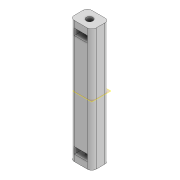
# Autodesk Inventor part: TopBottomConnector
Saved by Autodesk Inventor 2022 (Build 260153000, 153)
## iProperties
Created: 2022-10-26
Part Number: TopBottomConnector
Material: Generic
Document SubType Name: Modeling
Designer: MVeszpremi
Density: 1 g/cm^3
Appearance: Default
Author: MVeszpremi
Autodesk Inventor part; units mm, degrees
ref_plane "YZ Plane" through (0, 0, 0) normal (1, 0, 0) x (0, 1, 0)
ref_plane "XZ Plane" through (0, 0, 0) normal (0, 1, 0) x (-1, 0, 0)
ref_plane "XY Plane" through (0, 0, 0) normal (0, 0, 1) x (1, 0, 0)
sketch "Sketch1" plane through (0, 0, 0) normal (0, 1, 0) x (-1, 0, 0)
  line L0 (0, 0) -> (10, 0)
  line L1 (10, 0) -> (10, -8)
  line L2 (10, -8) -> (0, -8)
  line L3 (0, -8) -> (0, 0)
  circle A0 centre (5, -4) radius 1.5
  dimension "d0" = 10
  dimension "d1" = 8
  dimension "d2" = 3
  dimension "d11" = 5
  dimension "d12" = 4
  constraints: 8 end point, 2 parallel, 1 centre point, 1 horizontal, 1 perpendicular
  measures "d0" distance of L1.end L2.end
  measures "d1" distance of L0.end L1.end
  measures "d2" diameter of A0
  measures "d11" distance from line of A0.centre L1
  measures "d12" distance from line of L2 A0.centre
extrude "Extrusion1" add sketch "Sketch1" along normal blind 56
sketch "Sketch2" plane through (-10, 0, 0) normal (0, 0, 1) x (1, 0, 0)
  line L0 (2, 6) -> (8, 6)
  line L1 (8, 6) -> (8, 3)
  line L2 (8, 3) -> (2, 3)
  line L3 (2, 3) -> (2, 6)
  line L4 (0, 0) -> (0, 56) projected
  line L5 (0, 0) -> (10, 0) projected
  dimension "d5" = 6
  dimension "d6" = 2
  dimension "d7" = 3
  dimension "d8" = 3
  constraints: 8 end point, 2 parallel, 1 horizontal, 1 perpendicular
  measures "d5" distance of L0.start L0.end
  measures "d6" distance between parallel lines of L4 L3
  measures "d7" distance between parallel lines of L5 L2
  measures "d8" distance of L0.end L1.end
extrude "Extrusion2" cut sketch "Sketch2" against normal blind 61
ref_plane "Work Plane1" through (0, 28, 0) normal (0, 1, 0) x (1, 0, 0)
mirror "Mirror1" about plane through (0, 28, 0) normal (0, 1, 0) of "Extrusion2"
fillet "Fillet1" radius 2 4 edges at (-10, 28, 0) (0, 28, 0) (0, 28, -8) (-10, 28, -8)
body "Solid1"
